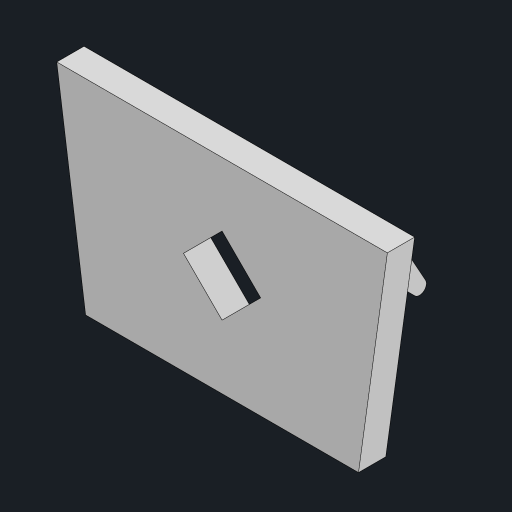
# Autodesk Inventor part: om_BackHolder_V4
Saved by Autodesk Inventor 2023 (Build 270158000, 158)
## iProperties
Created: 2022-07-14
Part Number: om_BackHolder_V4
Material: 一般
Document SubType Name: Modeling
Designer: legot
Density: 1 g/cm^3
Appearance: 既定
Author: legot
Autodesk Inventor part; units mm, degrees
ref_plane "XZ Plane" through (0, 0, 0) normal (0, 1, 0) x (-1, 0, 0)
ref_plane "XY Plane" through (0, 0, 0) normal (0, 0, 1) x (1, 0, 0)
sketch "スケッチ1" plane through (0, 0, 0) normal (0, 0, 1) x (1, 0, 0)
  line L0 (2.8284, 0) -> (0, -2.8284)
  line L1 (0, -2.8284) -> (-2.8284, 0)
  line L2 (-2.8284, 0) -> (0, 2.8284)
  line L3 (0, 2.8284) -> (2.8284, 0)
  line L4 (-12.1149, 7.5) -> (-10, -7.5)
  line L5 (10, -7.5) -> (-10, -7.5)
  line L6 (10, -7.5) -> (12.1149, 7.5)
  line L7 (12.1149, 7.5) -> (-12.1149, 7.5)
  point P0 (0, 0)
  point P1 (0, 7.5)
  point P2 (11.0574, 0)
  dimension "d10" = 24.2298
  dimension "d11" = 20
  dimension "d12" = 15
  dimension "d13" = 4
  constraints: 16 end point, 4 equal length, 3 vertical alignment, 2 horizontal alignment, 2 midpoint, 1 horizontal, 1 perpendicular
  measures "d10" distance of L6.end L4.start
  measures "d11" distance of L5.start L4.end
  measures "d12" distance between parallel lines of L7 L5
  measures "d13" distance of L2.end L0.start
extrude "押し出し1" add sketch "スケッチ1" against normal blind 2
ref_plane "作業平面1" through (10, 0, 0) normal (1, 0, 0) x (0, 1, 0)
sketch "スケッチ3" plane through (10, 0, 0) normal (1, 0, 0) x (0, 1, 0)
  line L0 (7.5, 0) -> (-7.5, 0) projected
  line L1 (7.5, 0) -> (7.5, -2) projected
  line L2 (-7.5, -2) -> (7.5, -2) projected
  line L3 (-7.5, 0) -> (-7.5, -2) projected
  line L4 (7.5, -2) -> (2.254, -4.912)
  line L5 (1.6578, -4.1213) -> (3.7791, -2)
  arc A0 (1.6578, -4.1213) -> (2.254, -4.912) centre (2.0114, -4.4749) ccw
  point P0 (0, 0)
  dimension "d17" = 0.5
  dimension "d18" = 45
  dimension "d19" = 6
  dimension "d25" = 3
  constraints: 4 end point, 2 point on circle, 2 tangent, 1 centre point, 1 point on line
  measures "d17" radius of A0
  measures "d18" angle of L2 L5
  measures "d19" distance of L1.end L4.end
  measures "d25" distance of L5.start L5.end
extrude "押し出し3" add sketch "スケッチ3" against normal blind 2 contours L4 A0 L5 L2
fillet "フィレット1" radius 1 2 edges at (10, 5.6396, -2) (8, 5.6396, -2)
fillet "フィレット2" radius 0.5 2 edges at (7.5, 3.7791, -2) (10.5, 3.7791, -2)
mirror "ミラー2" about plane through (0, 0, 0) normal (1, 0, 0) of "押し出し3", "フィレット1", "フィレット2"
